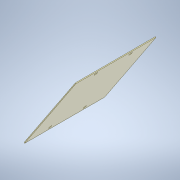
# Autodesk Inventor part: モーターガード
Saved by Autodesk Inventor 2020.2 (Build 242310000, 310)
## iProperties
Created: 2020-03-30
Part Number: モーターガード
Material: ポリプロピレン
Document SubType Name: Modeling
Designer: aoyama
Density: 0.899 g/cm^3
Appearance: 滑らか - 灰色
Author: aoyama
Autodesk Inventor part; units mm, degrees
ref_plane "YZ Plane" through (0, 0, 0) normal (1, 0, 0) x (0, 1, 0)
ref_plane "XZ Plane" through (0, 0, 0) normal (0, 1, 0) x (-1, 0, 0)
ref_plane "XY Plane" through (0, 0, 0) normal (0, 0, 1) x (1, 0, 0)
sketch "スケッチ1" plane through (0, 0, 0) normal (0, 0, 1) x (1, 0, 0)
  circle A0 centre (152.1225, -73.6752) radius 4
  line L0 (206.0478, 0.7) -> (205.7783, 0.7)
  circle A1 centre (152.1225, -73.6752) radius 4
  line L1 (206.0478, 0.7) -> (205.7783, 0.7)
  circle A2 centre (171.8792, -18.7507) radius 14
  circle A3 centre (-152.1225, 73.6752) radius 4
  line L2 (-206.0478, -0.7) -> (-205.7783, -0.7)
  circle A4 centre (-152.1225, 73.6752) radius 4
  line L3 (-206.0478, -0.7) -> (-205.7783, -0.7)
  circle A5 centre (-171.8792, 18.7507) radius 14
  line L4 (-152.1225, 73.6752) -> (-155.4555, 75.8868)
  line L5 (-155.4555, 75.8868) -> (-205.8083, 0)
  circle A6 centre (152.1225, -73.6752) radius 4
  line L6 (206.0478, 0.7) -> (205.7783, 0.7)
  circle A7 centre (171.8792, -18.7507) radius 14
  line L7 (250, 0) -> (156.4849, 0)
  line L8 (-250, 0) -> (-156.4849, 0)
  line L9 (-205.8083, -0.7) -> (-205.8083, 0)
  line L10 (-206.5583, -0.7) -> (-206.5583, 0.2262)
  line L11 (-206.5583, 0.2262) -> (-155.6658, 76.9264)
  line L12 (-155.6658, 76.9264) -> (-151.7078, 74.3002) construction
  line L13 (-155.4555, 75.8868) -> (-156.0804, 76.3015)
  line L14 (-205.8083, 0) -> (-206.4332, 0.4147)
  line L15 (-203.6688, 4.5809) -> (-203.0438, 4.1663)
  line L16 (-158.2199, 71.7205) -> (-158.8449, 72.1352)
  point P0 (0, 0)
  point P1 (205.8083, 0.7)
  point P2 (205.8083, 0.7)
  point P3 (205.8083, 0.7)
  dimension "d2" = 360
  dimension "d6" = 360
  dimension "d8" = 0.75
  dimension "d11" = 5
  dimension "d12" = 5
  dimension "d27" = 56.435
  constraints: 34 end point, 7 centre point, 7 point on line, 4 perpendicular, 3 horizontal, 1 collinear, 1 tangent, 53 other
  measures "d8" distance between parallel lines of L5 L11
  measures "d11" distance between parallel lines of L15 L14
  measures "d12" distance between parallel lines of L16 L13
  measures "d27" angle of L8 L5
extrude "押し出し1" add sketch "スケッチ1" along normal blind 78.6 contours L5 L16 L11 L13 | L5 L15 L11 L16 | L5 L14 L11 L15
sketch "スケッチ2" plane through (-206.4332, 0.4147, 0) normal (-0.8333, 0.5529, 0) x (0, 0, 1)
  line L0 (0, 91.0725) -> (0, 0) projected
  line L1 (0, 0) -> (78.6, 0) projected
  line L2 (78.6, 91.0725) -> (78.6, 0) projected
  line L3 (0, 91.0725) -> (78.6, 91.0725) projected
  line L4 (0, 86.0725) -> (78.6, 86.0725)
  line L5 (0, 5) -> (78.6, 5)
  line L6 (39.3, 91.0725) -> (39.3, 0)
  circle A0 centre (22.3, 5) radius 1.5
  circle A1 centre (56.3, 5) radius 1.5
  circle A2 centre (22.3, 86.0725) radius 1.5
  circle A3 centre (56.3, 86.0725) radius 1.5
  point P0 (0, 113.7886)
  dimension "d13" = 5
  dimension "d14" = 5
  dimension "d15" = 39.3
  dimension "d16" = 39.3
  dimension "d17" = 3
  dimension "d18" = 3
  dimension "d19" = 3
  dimension "d20" = 3
  dimension "d21" = 17
  dimension "d22" = 17
  dimension "d23" = 17
  dimension "d24" = 17
  constraints: 8 point on line, 6 end point, 4 centre point, 2 horizontal, 2 midpoint
  measures "d13" distance between parallel lines of L3 L4
  measures "d14" distance between parallel lines of L1 L5
  measures "d15" distance of L2.start L6.start
  measures "d16" distance of L0.start L6.start
  measures "d17" diameter of A0
  measures "d18" diameter of A1
  measures "d19" diameter of A2
  measures "d20" diameter of A3
  measures "d21" distance from line of L6 A0.centre
  measures "d22" distance from line of L6 A1.centre
  measures "d23" distance from line of L6 A2.centre
  measures "d24" distance from line of A3.centre L6
extrude "押し出し2" cut sketch "スケッチ2" against normal blind 10 contours A2 L4 | L4 A2 | A0 L5 | L5 A0 | A3 L4 | L4 A3 | A1 L5 | L5 A1
